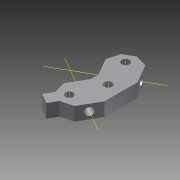
# Autodesk Inventor part: Vertex Bootm with foot
Saved by Autodesk Inventor 2013 (Build 170138000, 138)
## iProperties
Created: 2012-01-12
Part Number: Vertex Bootm with foot
Document SubType Name: Modeling
Designer: Nico
Density: 1 g/cm^3
Mass: 41.3247 g
Surface Area: 117.259 cm^2
Volume: 41.3247 cm^3
Material: Generic
Author: Nico
Autodesk Inventor part; units mm, degrees
ref_plane "YZ Plane" through (0, 0, 0) normal (1, 0, 0) x (0, 1, 0)
ref_plane "XZ Plane" through (0, 0, 0) normal (0, 1, 0) x (-1, 0, 0)
ref_plane "XY Plane" through (0, 0, 0) normal (0, 0, 1) x (1, 0, 0)
sketch "Sketch1" plane through (0, 0, 0) normal (0, 0, 1) x (1, 0, 0)
  line L0 (0, 0) -> (0, 34.48)
  line L1 (0, 34.48) -> (-11.25, 53.9656)
  line L2 (-11.25, 53.9656) -> (-23.6139, 57.2785)
  line L3 (-23.6139, 57.2785) -> (-33.9369, 51.3185)
  line L4 (-33.9369, 51.3185) -> (-37.2963, 38.7807)
  line L5 (-37.2963, 38.7807) -> (-27.1513, 21.2091)
  line L6 (-37.2963, -4.3007) -> (-33.9369, -16.8385)
  line L7 (-33.9369, -16.8385) -> (-23.6139, -22.7985)
  line L8 (-23.6139, -22.7985) -> (-11.25, -19.4856)
  line L9 (-11.25, -19.4856) -> (0, 0)
  line L10 (-37.2963, -4.3007) -> (-27.1513, 13.2709)
  line L11 (-27.1513, 13.2709) -> (-27.1513, 21.2091)
  circle A0 centre (-24.2754, 46.5042) radius 4
  circle A1 centre (-24.2754, -12.0242) radius 4
  line L12 (-33.9369, -16.8385) -> (-57.9984, -2.9465)
  line L13 (-33.9369, -16.8385) -> (-24.2152, 0)
  line L14 (-27.1513, 55.2361) -> (-5.625, 67.6643)
  line L15 (-23.6139, 57.2785) -> (-11.8125, 36.8379)
  circle A2 centre (-13.2, 17.24) radius 4
  dimension "d0" = 34.48
  dimension "d1" = 22.5
  dimension "d2" = 12.8
  dimension "d3" = 11.92
  dimension "d4" = 12.98
  dimension "d10" = 150
  dimension "d11" = 135
  dimension "d12" = 135
  dimension "d13" = 135
  dimension "d14" = 135
  dimension "d21" = 150
  dimension "d22" = 22.5
  dimension "d23" = 135
  dimension "d24" = 12.8
  dimension "d25" = 225
  dimension "d26" = 11.92
  dimension "d27" = 12.98
  dimension "d28" = 135
  dimension "d29" = 20.29
  dimension "d30" = 135
  dimension "d31" = 7.9382
  dimension "d32" = 9
  dimension "d33" = 9
  dimension "d34" = 5.96
  dimension "d35" = 5.96
  dimension "d36" = 8
  dimension "d37" = 8
  dimension "d38" = 13.2
  dimension "d39" = 8
  constraints: 32 end point, 5 perpendicular, 3 centre point, 2 parallel, 1 point on line, 1 vertical
  measures "d0" distance of L0.start L0.end
  measures "d1" distance of L0.end L1.end
  measures "d2" distance of L1.end L2.end
  measures "d3" distance of L2.end L3.end
  measures "d4" distance of L3.end L4.end
  measures "d10" angle of L0 L1
  measures "d11" angle of L1 L2
  measures "d12" angle of L3 L2
  measures "d13" angle of L4 L3
  measures "d14" angle of L5 L4
  measures "d21" angle of L9 L0
  measures "d22" distance of L8.end L0.start
  measures "d23" angle of L8 L9
  measures "d24" distance of L7.end L8.end
  measures "d26" distance of L6.end L7.end
  measures "d27" distance of L6.start L6.end
  measures "d28" angle of L7 L6
  measures "d29" distance of L6.start L10.end
  measures "d30" angle of L6 L10
  measures "d31" distance of L10.end L5.end
  measures "d32" distance from line of A0.centre L3
  measures "d33" distance from line of L7 A1.centre
  measures "d34" distance from line of L13 A1.centre
  measures "d35" distance from line of L15 A0.centre
  measures "d36" diameter of A0
  measures "d37" diameter of A1
  measures "d38" distance from line of A2.centre L0
  measures "d39" diameter of A2
extrude "Extrusion1" add sketch "Sketch1" along normal blind 14
sketch "Sketch2" plane through (0, 34.48, 14) normal (0.866, 0.5, 0) x (0, 0, -1)
  line L0 (0, 22.5) -> (0, 0) projected
  line L1 (14, 0) -> (0, 0) projected
  line L2 (14, 22.5) -> (0, 22.5) projected
  circle A0 centre (7, 11.25) radius 4
  point P0 (14, -29.8606)
  dimension "d42" = 22.5
  dimension "d43" = 11.25
  dimension "d44" = 7
  dimension "d52" = 8
  constraints: 1 centre point
  measures "d42" distance between parallel lines of L1 L2
  measures "d43" distance from line of A0.centre L2
  measures "d44" distance from line of A0.centre L0
  measures "d52" diameter of A0
extrude "Extrusion2" cut sketch "Sketch2" against normal blind 40
sketch "Sketch3" plane through (-11.25, -19.4856, 14) normal (0.866, -0.5, 0) x (0, 0, -1)
  line L0 (14, 0) -> (14, 22.5) projected
  line L1 (14, 22.5) -> (0, 22.5) projected
  circle A0 centre (7, 11.25) radius 4
  line L2 (14, -9.051) -> (0, -9.051) projected
  dimension "d47" = 8
  dimension "d48" = 11.25
  dimension "d49" = 7
  dimension "d64" = 20.301
  constraints: 1 centre point
  measures "d47" diameter of A0
  measures "d48" distance from line of A0.centre L1
  measures "d49" distance from line of A0.centre L0
  measures "d64" distance from line of L2 A0.centre
extrude "Extrusion3" cut sketch "Sketch3" against normal blind 40
sketch "Sketch5" plane through (-33.9369, -16.8385, 0) normal (-0.5, -0.866, 0) x (0.866, -0.5, 0)
  line L0 (11.92, 0) -> (0, 0)
  line L1 (0, 0) -> (0, 14)
  line L2 (0, 14) -> (11.92, 14)
  line L3 (11.92, 14) -> (11.92, 0)
  point P0 (20.971, 0)
  constraints: 8 end point, 2 parallel, 1 horizontal, 1 perpendicular
extrude "Extrusion4" add sketch "Sketch5" along normal blind 10
body "Solid1"
